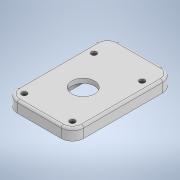
# Autodesk Inventor part: SwitchHolder
Saved by Autodesk Inventor 2022 (Build 260153000, 153)
## iProperties
Created: 2023-04-13
Part Number: SwitchHolder
Material: Generic
Document SubType Name: Modeling
Designer: richb366163
Density: 1 g/cm^3
Appearance: Default
Author: richb366163
Autodesk Inventor part; units mm, degrees
ref_plane "YZ Plane" through (0, 0, 0) normal (1, 0, 0) x (0, 1, 0)
ref_plane "XZ Plane" through (0, 0, 0) normal (0, 1, 0) x (-1, 0, 0)
ref_plane "XY Plane" through (0, 0, 0) normal (0, 0, 1) x (1, 0, 0)
sketch "Sketch1" plane through (0, 0, 0) normal (0, 1, 0) x (-1, 0, 0)
  circle A0 centre (0, 0) radius 5.715
  line L0 (0, 0) -> (8.382, 0)
  line L1 (8.382, 0) -> (8.382, 14.3891)
  line L2 (8.382, 14.3891) -> (0, 14.3891)
  line L3 (0, 14.3891) -> (0, 0)
  line L4 (8.382, 14.3891) -> (-8.382, 14.3891)
  line L5 (-8.382, 14.3891) -> (-8.382, -14.3891)
  line L6 (-8.382, -14.3891) -> (8.382, -14.3891)
  line L7 (8.382, -14.3891) -> (8.382, 14.3891)
  line L8 (8.382, 14.3891) -> (13.462, 14.3891)
  line L9 (13.462, 14.3891) -> (13.462, 19.4691)
  line L10 (13.462, 19.4691) -> (8.382, 19.4691)
  line L11 (8.382, 19.4691) -> (8.382, 14.3891)
  line L12 (-8.382, -14.3891) -> (-13.462, -14.3891)
  line L13 (-13.462, -14.3891) -> (-13.462, -19.4691)
  line L14 (-13.462, -19.4691) -> (-8.382, -19.4691)
  line L15 (-8.382, -19.4691) -> (-8.382, -14.3891)
  line L16 (13.462, 19.4691) -> (-13.462, 19.4691)
  line L17 (-13.462, 19.4691) -> (-13.462, -19.4691)
  line L18 (-13.462, -19.4691) -> (13.462, -19.4691)
  line L19 (13.462, -19.4691) -> (13.462, 19.4691)
  circle A1 centre (13.462, 19.4691) radius 1.5
  circle A2 centre (-13.462, 19.4691) radius 1.5
  circle A3 centre (-13.462, -19.4691) radius 1.5
  circle A4 centre (13.462, -19.4691) radius 1.5
  line L20 (13.462, 24.5491) -> (-18.542, 24.5491)
  line L21 (-18.542, 24.5491) -> (-18.542, -19.4691)
  line L22 (18.542, 19.4691) -> (18.542, -24.5491)
  line L23 (18.542, -24.5491) -> (-13.462, -24.5491)
  line L24 (13.462, 19.4691) -> (18.542, 19.4691)
  line L25 (18.542, 19.4691) -> (18.542, 24.5491)
  line L26 (18.542, 24.5491) -> (13.462, 24.5491)
  line L27 (13.462, 24.5491) -> (13.462, 19.4691)
  line L28 (-18.542, -19.4691) -> (-13.462, -19.4691)
  line L29 (-13.462, -19.4691) -> (-13.462, -24.5491)
  line L30 (-13.462, -24.5491) -> (-18.542, -24.5491)
  line L31 (-18.542, -24.5491) -> (-18.542, -19.4691)
  line L32 (-18.542, -24.5491) -> (18.542, -24.5491)
  line L33 (18.542, -24.5491) -> (18.542, -32.1691)
  line L34 (18.542, -32.1691) -> (-18.542, -32.1691)
  line L35 (-18.542, -32.1691) -> (-18.542, -24.5491)
  point P0 (0, 14.3891)
  point P1 (18.542, -24.5491)
  dimension "d0" = 11.43
  dimension "d1" = 8.382
  dimension "d2" = 14.3891
  dimension "d3" = 16.764
  dimension "d4" = 28.7782
  dimension "d5" = 5.08
  dimension "d6" = 5.08
  dimension "d7" = 5.08
  dimension "d8" = 5.08
  dimension "d9" = 3
  dimension "d10" = 3
  dimension "d11" = 3
  dimension "d12" = 3
  dimension "d13" = 5.08
  dimension "d14" = 5.08
  dimension "d22" = 7.62
  constraints: 72 end point, 16 parallel, 9 perpendicular, 8 horizontal, 5 centre point, 5 coincident, 1 collinear, 2 other
  measures "d0" diameter of A0
  measures "d1" distance of L2.end L1.end
  measures "d2" distance of L1.end L0.end
  measures "d3" distance of L6.end L5.end
  measures "d4" distance of L5.end L4.end
  measures "d5" distance of L10.end L9.end
  measures "d6" distance of L9.end L8.end
  measures "d7" distance of L14.end L13.end
  measures "d8" distance of L12.end L13.end
  measures "d9" diameter of A1
  measures "d10" diameter of A2
  measures "d11" diameter of A3
  measures "d12" diameter of A4
  measures "d13" distance between parallel lines of L16 L20
  measures "d14" distance between parallel lines of L19 L22
  measures "d22" distance of L32.end L33.end
extrude "Extrusion1" add sketch "Sketch1" along normal blind 3.81 contours L1 L8 L19 A4 L18 L15 L6 L7 | L4 L5 L12 L17 A2 L16 L11 L2 | L11 L10 A1 L9 L8 | L9 A1 L24 L22 L23 L29 A3 L14 L18 A4 L19 | L16 A2 L17 L13 A3 L28 L21 L20 L27 A1 L10 | L15 L14 A3 L13 L12 | A1 L27 L26 L25 L24 | A3 L29 L30 L31 L28 | L33 L34 L35 L30 L23
sketch "Sketch2" plane through (0, 3.81, 0) normal (0, 1, 0) x (1, 0, 0)
  circle A0 centre (0, 0) radius 6.35
  line L0 (-18.542, -24.5491) -> (18.542, -24.5491) projected
  circle A1 centre (13.462, 19.4691) radius 1.5 projected
  line L1 (-8.382, -14.3891) -> (-8.382, 14.3891) projected
  line L2 (-8.382, 14.3891) -> (8.382, 14.3891) projected
  line L3 (8.382, 14.3891) -> (8.382, -14.3891) projected
  line L4 (8.382, -14.3891) -> (-8.382, -14.3891) projected
  circle A2 centre (13.462, -19.4691) radius 1.5 projected
  circle A3 centre (-13.462, 19.4691) radius 1.5 projected
  circle A4 centre (-13.462, -19.4691) radius 1.5 projected
  line L5 (-18.542, 32.1691) -> (-18.542, -24.5491) projected
  line L6 (18.542, -24.5491) -> (18.542, 32.1691) projected
  line L7 (18.542, 32.1691) -> (-18.542, 32.1691) projected
  dimension "d17" = 12.7
  constraints: 1 centre point, 1 coincident
  measures "d17" diameter of A0
extrude "Extrusion2" add sketch "Sketch2" along normal blind 2.54 contours L5 L7 L6 L0 | L1 L2 L3 L4
fillet "Fillet1" radius 6.35 4 edges at (-18.542, 3.175, 24.5491) (18.542, 3.175, 24.5491) (18.542, 3.175, -32.1691) (-18.542, 3.175, -32.1691)
fillet "Fillet2" radius 1.27 3 edges at (16.6821, 6.35, 22.6892) (-16.6821, 6.35, 22.6892) (0, 6.35, 24.5491)
body "Solid1"
